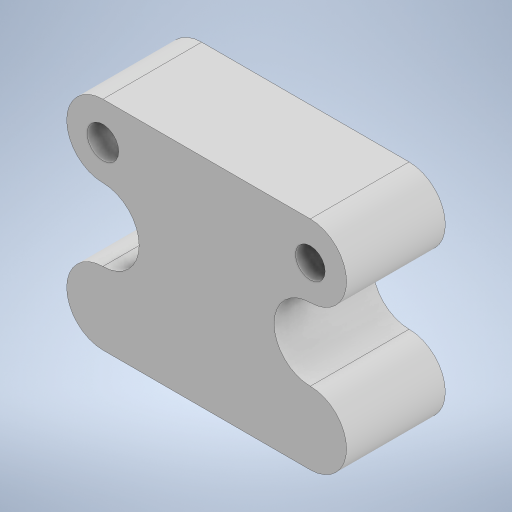
# Autodesk Inventor part: Zipperteethv7
Saved by Autodesk Inventor 2023.1 (Build 271208000, 208)
## iProperties
Created: 2022-11-10
Part Number: Zipperteethv7
Material: Generic
Document SubType Name: Modeling
Designer: Grimm
Density: 1 g/cm^3
Appearance: Default
Author: Grimm
Autodesk Inventor part; units mm, degrees
ref_plane "YZ Plane" through (0, 0, 0) normal (1, 0, 0) x (0, 1, 0)
ref_plane "XZ Plane" through (0, 0, 0) normal (0, 1, 0) x (-1, 0, 0)
ref_plane "XY Plane" through (0, 0, 0) normal (0, 0, 1) x (1, 0, 0)
sketch "Sketch1" plane through (0, 0, 0) normal (0, 0, 1) x (1, 0, 0)
  line L0 (-13.9136, 8.9772) -> (28.0864, 8.9772)
  line L1 (28.0864, 8.9772) -> (28.0864, -13.0228)
  line L2 (28.0864, -13.0228) -> (-13.9136, -13.0228)
  line L3 (-13.9136, -13.0228) -> (-13.9136, 8.9772)
  point P0 (0, 0)
  dimension "d0" = 42
  dimension "d1" = 22
  constraints: 8 end point, 2 parallel, 1 horizontal, 1 perpendicular
  measures "d0" distance of L1.end L2.end
  measures "d1" distance of L0.end L1.end
extrude "Extrusion1" add sketch "Sketch1" along normal blind 10
sketch "Sketch2" plane through (0, 0, 10) normal (0, 0, 1) x (1, 0, 0)
  line L0 (-13.9136, -13.0228) -> (28.0864, -13.0228) projected
  arc A0 (-3.4134, -5.6894) -> (-3.4136, -13.0228) centre (-3.4136, -9.3561) ccw
  arc A1 (-3.4134, -5.6894) -> (-3.4134, 1.6439) centre (-3.4133, -2.0228) ccw
  arc A2 (17.5864, -13.0228) -> (17.5862, -5.6894) centre (17.5864, -9.3561) ccw
  arc A3 (17.5862, 1.6439) -> (17.5862, -5.6894) centre (17.586, -2.0228) ccw
  line L1 (-3.4136, -13.0228) -> (17.5864, -13.0228)
  line L2 (-3.4135, 8.9772) -> (17.5865, 8.9772)
  line L3 (28.0864, 8.9772) -> (-13.9136, 8.9772) projected
  line L4 (-3.4133, -2.0228) -> (-3.4136, -9.3561) construction
  line L5 (17.5864, -9.3561) -> (17.586, -2.0228) construction
  arc A4 (-3.4135, 8.9772) -> (-3.4134, 1.6439) centre (-3.4136, 5.3106) ccw
  arc A5 (17.5862, 1.6439) -> (17.5865, 8.9772) centre (17.5864, 5.3106) ccw
  line L6 (-3.4133, -2.0228) -> (-13.9136, -2.0228) construction
  line L7 (17.586, -2.0228) -> (28.0864, -2.0228) construction
  line L8 (28.0864, -13.0228) -> (28.0864, 8.9772) construction
  line L9 (-13.9136, 8.9772) -> (-13.9136, -13.0228) projected
  line L10 (-7.0803, -9.356) -> (-13.9136, -9.356) construction
  line L11 (21.2531, -9.356) -> (28.0864, -9.356) construction
  line L12 (-13.9136, -13.0228) -> (28.0864, -13.0228)
  line L13 (28.0864, -13.0228) -> (28.0864, 8.9772)
  line L14 (28.0864, 8.9772) -> (-13.9136, 8.9772)
  line L15 (-13.9136, 8.9772) -> (-13.9136, -13.0228)
  line L16 (-7.0803, 5.3105) -> (-13.9136, 5.3105) construction
  line L17 (21.2531, 5.3105) -> (28.0864, 5.3105) construction
  point P0 (0, 0)
  point P1 (17.8152, 8.9772)
  point P2 (-3.4136, 8.9772)
  point P3 (-3.4136, 8.9772)
  dimension "d4" = 21
  dimension "d5" = 22
  dimension "d17" = 21
  constraints: 28 end point, 16 point on circle, 10 point on line, 8 tangent, 6 centre point, 5 collinear, 5 equal radius, 4 midpoint, 4 perpendicular, 2 horizontal
  measures "d4" distance of L1.end L1.start
  measures "d5" distance between parallel lines of L0 L2
  measures "d17" distance of L2.end L2.start
extrude "Extrusion2" cut sketch "Sketch2" against normal blind 10 contours L9 L3 A4 A1 A0 L0 | A2 A3 A5 L3 L13 L0
sketch "Sketch3" plane through (0, 0, 10) normal (0, 0, 1) x (1, 0, 0)
  arc A0 (-3.4134, -5.6894) -> (-3.4134, 1.6439) centre (-3.4133, -2.0228) ccw construction
  line L0 (-7.2207, -5.6893) -> (3.1864, -5.6897) construction
  line L1 (20.3968, -5.6893) -> (9.686, -5.6898) construction
  arc A1 (-3.4134, -5.6894) -> (-3.4136, -13.0228) centre (-3.4136, -9.3561) ccw construction
  arc A2 (-3.4134, -5.6894) -> (-3.4134, 1.6439) centre (-3.4133, -2.0228) ccw construction
  arc A3 (17.5864, -13.0228) -> (17.5862, -5.6894) centre (17.5864, -9.3561) ccw construction
  arc A4 (17.5862, 1.6439) -> (17.5862, -5.6894) centre (17.586, -2.0228) ccw construction
  line L2 (-3.4137, -11.3763) -> (-3.4129, 5.1845) construction
  line L3 (17.5866, -13.0364) -> (17.5857, 5.1238) construction
  arc A5 (17.5862, 1.6439) -> (17.5862, -5.6894) centre (17.586, -2.0228) ccw construction
  point P0 (0, 0)
  constraints: 8 end point, 4 coincident, 4 tangent, 2 perpendicular, 2 point on line
hole "Hole1" at (17.5857, 5.1238, 10) direction (0, 0, -1) diameter 3 end through all
hole "Hole2" at (-3.4129, 5.1845, 10) direction (0, 0, -1) diameter 3.2 end through all
body "Solid1"
